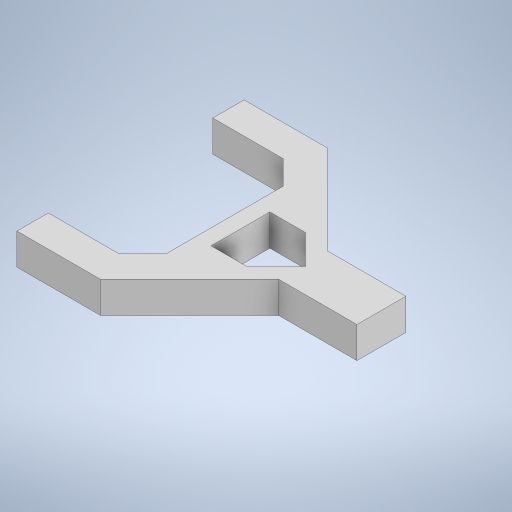
# Autodesk Inventor part: bottom
Saved by Autodesk Inventor 2023.1 (Build 271208000, 208)
## iProperties
Created: 2023-11-14
Part Number: bottom
Material: Generic
Document SubType Name: Modeling
Designer: zavrel
Density: 1 g/cm^3
Appearance: Default
Author: zavrel
Autodesk Inventor part; units mm, degrees
ref_plane "YZ Plane" through (0, 0, 0) normal (1, 0, 0) x (0, 1, 0)
ref_plane "XZ Plane" through (0, 0, 0) normal (0, 1, 0) x (-1, 0, 0)
ref_plane "XY Plane" through (0, 0, 0) normal (0, 0, 1) x (1, 0, 0)
sketch "Sketch1" plane through (0, 0, 0) normal (0, 1, 0) x (-1, 0, 0)
  line L0 (0, 0) -> (0, 12.5)
  line L1 (0, 12.5) -> (40, 12.5)
  line L2 (40, 12.5) -> (85.5, 58)
  line L3 (72, 0) -> (72, 15)
  line L4 (72, 15) -> (53.8137, 15)
  line L5 (53.8137, 15) -> (38.8137, 0)
  line L6 (95.3823, 56.5685) -> (38.8137, 0) construction
  line L7 (80, 29.8726) -> (92.1274, 42)
  line L8 (92.1274, 42) -> (128.1464, 42)
  line L9 (128.1464, 42) -> (128.1464, 58)
  line L10 (128.1464, 58) -> (85.5, 58)
  line L11 (80, 29.8726) -> (80, 0)
  line L12 (0, 0) -> (142.506, 0) construction
  line L13 (0, 0) -> (0, -12.5)
  line L14 (0, -12.5) -> (40, -12.5)
  line L15 (40, -12.5) -> (85.5, -58)
  line L16 (72, 0) -> (72, -15)
  line L17 (72, -15) -> (53.8137, -15)
  line L18 (53.8137, -15) -> (38.8137, 0)
  line L19 (95.3823, -56.5685) -> (38.8137, 0) construction
  line L20 (80, -29.8726) -> (92.1274, -42)
  line L21 (92.1274, -42) -> (128.1464, -42)
  line L22 (128.1464, -42) -> (128.1464, -58)
  line L23 (128.1464, -58) -> (85.5, -58)
  line L24 (80, -29.8726) -> (80, 0)
  point P0 (128.1464, -50)
  point P1 (128.1464, 50)
  dimension "d2" = 40
  dimension "d7" = 45
  dimension "d9" = 8
  dimension "d12" = 16
  dimension "d14" = 30
  dimension "d15" = 25
  dimension "d16" = 8
  dimension "d17" = 100
  dimension "d20" = 16
  constraints: 50 end point, 10 symmetric about line, 4 perpendicular, 3 vertical, 2 horizontal, 2 midpoint, 1 parallel
  measures "d2" distance of L0.end L1.end
  measures "d7" angle of L2 L0
  measures "d9" distance between parallel lines of L5 L2
  measures "d12" distance of L8.end L9.end
  measures "d14" distance between parallel lines of L4 L17
  measures "d15" distance between parallel lines of L14 L1
  measures "d16" distance between parallel lines of L11 L3
  measures "d17" distance of point (128.146, -50) point (128.146, 50)
  measures "d20" distance between parallel lines of L2 L7
extrude "Extrusion1" add sketch "Sketch1" along normal blind 16
body "Solid1"
